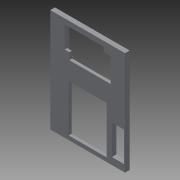
# Autodesk Inventor part: DisplayBottom2
Saved by Autodesk Inventor 2014 SP1 (Build 180222100, 222)
## iProperties
Created: 2014-03-24
Part Number: DisplayBottom2
Material: Generic
Document SubType Name: Modeling
Designer: patrigg
Density: 1 g/cm^3
Appearance: Default
Author: patrigg
Autodesk Inventor part; units mm, degrees
ref_plane "YZ Plane" through (0, 0, 0) normal (1, 0, 0) x (0, 1, 0)
ref_plane "XZ Plane" through (0, 0, 0) normal (0, 1, 0) x (-1, 0, 0)
ref_plane "XY Plane" through (0, 0, 0) normal (0, 0, 1) x (1, 0, 0)
sketch "Sketch2" plane through (0, 0, 0) normal (0, 1, 0) x (-1, 0, 0)
  line L0 (-32.5, -45) -> (32.5, -45)
  line L1 (32.5, -45) -> (32.5, 45)
  line L2 (32.5, 45) -> (-32.5, 45)
  line L3 (-32.5, 45) -> (-32.5, -45)
  line L4 (-32.5, -45) -> (32.5, 45) construction
  line L5 (32.5, -45) -> (-32.5, 45) construction
  point P0 (0, 0)
  dimension "d0" = 65
  dimension "d1" = 90
  constraints: 12 end point, 2 midpoint, 2 parallel, 1 horizontal, 1 perpendicular
  measures "d0" distance of L2.end L1.end
  measures "d1" distance of L1.end L0.end
extrude "Extrusion1" add sketch "Sketch2" along normal blind 4
sketch "Sketch3" plane through (0, 4, 0) normal (0, 1, 0) x (1, 0, 0)
  line L0 (32.5, 45) -> (-32.5, 45) projected
  line L1 (-19, -9.5) -> (19, -9.5)
  line L2 (19, -9.5) -> (19, 43)
  line L3 (19, 43) -> (-19, 43)
  line L4 (-19, 43) -> (-19, -9.5)
  line L5 (-19, -9.5) -> (19, 43) construction
  line L6 (19, -9.5) -> (-19, 43) construction
  line L7 (-32.5, 45) -> (-32.5, -45) projected
  point P0 (0, 0)
  point P1 (0, 16.75)
  dimension "d4" = 38
  dimension "d5" = 52.5
  dimension "d6" = 2
  dimension "d111" = 13.5
  constraints: 12 end point, 2 midpoint, 2 parallel, 1 horizontal, 1 perpendicular
  measures "d4" distance of L3.end L2.end
  measures "d5" distance of L2.end L1.end
  measures "d6" distance between parallel lines of L0 L3
  measures "d111" distance between parallel lines of L4 L7
extrude "Extrusion2" cut sketch "Sketch3" against normal blind 1.5
sketch "Sketch4" plane through (0, 2.5, 0) normal (0, 1, 0) x (1, 0, 0)
  line L0 (19, -9.5) -> (-19, -9.5) projected
  line L1 (19, 43) -> (19, -9.5) projected
  line L2 (-19, 43) -> (19, 43) projected
  line L3 (-19, -9.5) -> (-19, 43) projected
  line L4 (-16.5, 41.5) -> (16.5, 41.5)
  line L5 (16.5, 41.5) -> (16.5, 0.5)
  line L6 (16.5, 0.5) -> (-16.5, 0.5)
  line L7 (-16.5, 0.5) -> (-16.5, 41.5)
  line L8 (-16.5, 41.5) -> (16.5, 0.5) construction
  line L9 (16.5, 41.5) -> (-16.5, 0.5) construction
  point P0 (0, 0)
  point P1 (0, 21)
  dimension "d9" = 10
  dimension "d10" = 1.5
  dimension "d11" = 2.5
  dimension "d12" = 2.5
  constraints: 12 end point, 2 midpoint, 2 parallel, 1 horizontal, 1 perpendicular
  measures "d9" distance between parallel lines of L0 L6
  measures "d10" distance between parallel lines of L2 L4
  measures "d11" distance between parallel lines of L1 L5
  measures "d12" distance between parallel lines of L3 L7
extrude "Extrusion3" cut sketch "Sketch4" against normal blind 2.5 contours L4 L5 L6 L7
sketch "Sketch5" plane through (0, 4, 0) normal (0, 1, 0) x (1, 0, 0)
  line L0 (19, 43) -> (19, -9.5) projected
  line L1 (19, -9.5) -> (-19, -9.5) projected
  line L2 (-19, -9.5) -> (-19, 43) projected
  line L3 (-17, -15.5) -> (-17, -9.5)
  line L4 (17, -15.5) -> (17, -9.5)
  line L5 (32.5, 45) -> (-32.5, 45) projected
  line L6 (-17, -15.5) -> (17, -15.5)
  point P0 (0, 0)
  dimension "d18" = 2
  dimension "d19" = 2
  constraints: 6 end point, 2 perpendicular, 2 point on line, 1 parallel
  measures "d18" distance between parallel lines of L3 L2
  measures "d19" distance between parallel lines of L0 L4
extrude "Extrusion4" cut sketch "Sketch5" against normal blind 0.25
sketch "Sketch12" plane through (0, 4, 0) normal (0, 1, 0) x (1, 0, 0)
  line L0 (17, -15.5) -> (-17, -15.5) projected
  line L1 (-32.5, -45) -> (32.5, -45) projected
  line L2 (-20, -40.5) -> (20, -40.5)
  line L3 (20, -40.5) -> (20, -15.5)
  line L4 (20, -15.5) -> (-20, -15.5)
  line L5 (-20, -15.5) -> (-20, -40.5)
  line L6 (-20, -40.5) -> (20, -15.5) construction
  line L7 (20, -40.5) -> (-20, -15.5) construction
  line L8 (-19, -9.5) -> (-19, 43) projected
  point P0 (0, 0)
  point P1 (0, -28)
  point P2 (0, -28)
  point P3 (0, -45)
  dimension "d58" = 40
  dimension "d59" = 25
  dimension "d112" = 1
  constraints: 12 end point, 4 midpoint, 2 parallel, 1 collinear, 1 horizontal, 1 perpendicular
  measures "d58" distance of L4.end L3.end
  measures "d59" distance of L3.end L2.end
  measures "d112" distance between parallel lines of L5 L8
extrude "Extrusion10" cut sketch "Sketch12" against normal blind 4
sketch "Sketch16" plane through (0, 3.75, 0) normal (0, 1, 0) x (1, 0, 0)
  line L0 (-17, -15.5) -> (-17, -9.5) projected
  line L1 (17, -15.5) -> (-17, -15.5) projected
  line L2 (17, -15.5) -> (16, -15.5) projected
  line L3 (17, -9.5) -> (17, -15.5) projected
  line L4 (-17, -9.5) -> (17, -9.5) projected
  point P0 (0, 0)
extrude "Extrusion15" cut sketch "Sketch16" against normal up to next
sketch "Sketch18" plane through (20, 4, 15.5) normal (-1, 0, 0) x (0, 0, 1)
  line L0 (0, 0) -> (25, 0) projected
  line L1 (25, -4) -> (21, -4)
  line L2 (21, -4) -> (21, -1.8)
  line L3 (21, -1.8) -> (25, -1.8)
  line L4 (25, -1.8) -> (25, -4)
  point P0 (-15.5, -4)
  dimension "d88" = 4
  dimension "d89" = 1.8
  constraints: 8 end point, 2 parallel, 1 horizontal, 1 perpendicular
  measures "d88" distance of L2.end L3.end
  measures "d89" distance between parallel lines of L3 L0
extrude "Extrusion17" add sketch "Sketch18" along normal blind 6
sketch "Sketch20" plane through (-20, 4, 40.5) normal (1, 0, 0) x (0, 0, -1)
  line L0 (0, 0) -> (25, 0) projected
  line L1 (25, -4) -> (19, -4)
  line L2 (19, -4) -> (19, -1.8)
  line L3 (19, -1.8) -> (25, -1.8)
  line L4 (25, -1.8) -> (25, -4)
  point P0 (40.5, -4)
  dimension "d96" = 6
  dimension "d97" = 1.8
  constraints: 8 end point, 2 parallel, 1 horizontal, 1 perpendicular
  measures "d96" distance of L2.end L3.end
  measures "d97" distance between parallel lines of L3 L0
extrude "Extrusion19" add sketch "Sketch20" along normal blind 4
sketch "Sketch21" plane through (-17, 2.5, 9.5) normal (0, 0, 1) x (1, 0, 0)
  line L0 (34, 0) -> (0, 0) projected
  line L1 (0, 0) -> (0, -2.5) projected
  line L2 (34, -2.5) -> (0, -2.5) projected
  line L3 (34, 0) -> (34, -2.5) projected
  point P0 (17, -2.5)
extrude "Extrusion20" add sketch "Sketch21" along normal up to surface (6 mm away)
sketch "Sketch22" plane through (0, 0, 0) normal (0, -1, 0) x (1, 0, 0)
  line L0 (32.5, 45) -> (32.5, -45) projected
  line L1 (-32.5, 45) -> (32.5, 45) projected
  line L2 (31.5, -39) -> (21, -39)
  line L3 (21, -39) -> (21, -13)
  line L4 (21, -13) -> (31.5, -13)
  line L5 (31.5, -13) -> (31.5, -39)
  point P0 (0, 0)
  dimension "d102" = 1
  dimension "d103" = 10.5
  dimension "d107" = 84
  dimension "d110" = 26
  constraints: 8 end point, 2 parallel, 1 horizontal, 1 perpendicular
  measures "d102" distance between parallel lines of L5 L0
  measures "d103" distance between parallel lines of L3 L5
  measures "d107" distance between parallel lines of L2 L1
  measures "d110" distance between parallel lines of L4 L2
extrude "Extrusion21" cut sketch "Sketch22" against normal up to next
body "Solid1"
